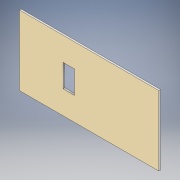
# Autodesk Inventor part: Window Gyp Board
Saved by Autodesk Inventor 2017 (Build 210142000, 142)
## iProperties
Created: 2017-05-30
Part Number: Window Gyp Board
Material: Generic
Document SubType Name: Modeling
Designer: cas7
Density: 1 g/cm^3
Appearance: Default
Mass: 11614.3 g
Surface Area: 15309.6 cm^2
Volume: 11614.3 cm^3
Author: cas7
Autodesk Inventor part; units mm, degrees
ref_plane "YZ Plane" through (0, 0, 0) normal (1, 0, 0) x (0, 1, 0)
ref_plane "XZ Plane" through (0, 0, 0) normal (0, 1, 0) x (-1, 0, 0)
ref_plane "XY Plane" through (0, 0, 0) normal (0, 0, 1) x (1, 0, 0)
sketch "Sketch1" plane through (0, 0, 0) normal (0, 0, 1) x (1, 0, 0)
  line L0 (0, 0) -> (1219.2, 0)
  line L1 (1219.2, 0) -> (1219.2, 609.6)
  line L2 (1219.2, 609.6) -> (0, 609.6)
  line L3 (0, 609.6) -> (0, 0)
  dimension "d0" = 1219.2
  dimension "d1" = 609.6
  constraints: 8 end point, 2 parallel, 1 horizontal, 1 perpendicular
  measures "d0" distance of L2.end L1.end
  measures "d1" distance of L1.end L0.end
extrude "Extrusion1" add sketch "Sketch1" along normal blind 15.875
sketch "Sketch6" plane through (0, 0, 15.875) normal (0, 0, 1) x (1, 0, 0)
  line L0 (482.6, 404.8) -> (382.6, 404.8)
  line L1 (482.6, 204.8) -> (382.6, 204.8)
  line L2 (382.6, 204.8) -> (382.6, 404.8)
  line L3 (482.6, 404.8) -> (482.6, 204.8)
  constraints: 8 end point, 1 parallel, 1 vertical
extrude "Extrusion5" cut sketch "Sketch6" against normal blind 90
body "Solid1"
